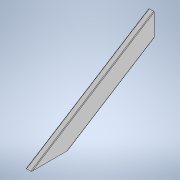
# Autodesk Inventor part: VerstaerkungHintenSchraeg
Saved by Autodesk Inventor 2020.3 (Build 243373010, 373A)
## iProperties
Created: 2021-02-13
Part Number: VerstaerkungHintenSchraeg
Material: Generisch
Document SubType Name: Modeling
Designer: Stefan
Density: 1 g/cm^3
Appearance: Vorgabe
Author: Stefan
Autodesk Inventor part; units mm, degrees
ref_plane "YZ Plane" through (0, 0, 0) normal (1, 0, 0) x (0, 1, 0)
ref_plane "XZ Plane" through (0, 0, 0) normal (0, 1, 0) x (-1, 0, 0)
ref_plane "XY Plane" through (0, 0, 0) normal (0, 0, 1) x (1, 0, 0)
sketch "Skizze1" plane through (0, 0, 0) normal (1, 0, 0) x (0, 1, 0)
  line L0 (384.3381, -178.6102) -> (384.3381, -313.6102)
  line L1 (384.3381, -313.6102) -> (584.3932, -631.3447)
  line L2 (584.3932, -631.3447) -> (669.3932, -631.3447)
  line L3 (669.3932, -631.3447) -> (384.3381, -178.6102)
  point P0 (0, 0)
  dimension "d0" = 135
  dimension "d1" = 85
  dimension "d2" = 535
  dimension "d3" = 375.4694
  constraints: 8 end point, 1 parallel, 1 perpendicular, 1 vertical
  measures "d0" distance of L0.start L0.end
  measures "d1" distance of L1.end L2.end
  measures "d2" distance of L2.end L0.start
  measures "d3" distance of L0.end L1.end
extrude "Extrusion1" add sketch "Skizze1" along normal blind 20
fillet "Rundung1" radius 2 4 edges at (20, 526.8656, -404.9774) (0, 526.8656, -404.9774) (20, 484.3656, -472.4774) (0, 484.3656, -472.4774)
